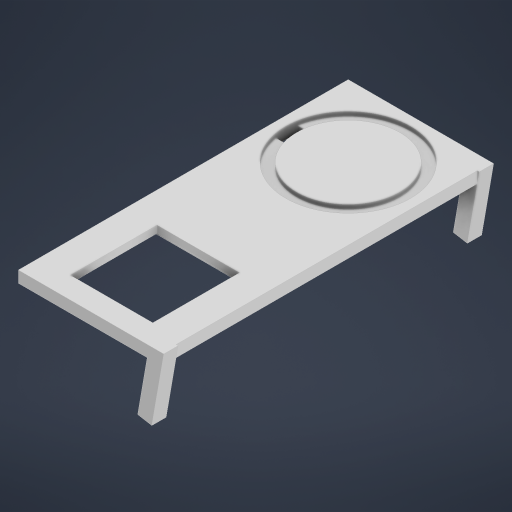
# Autodesk Inventor part: ViesCooleHouder
Saved by Autodesk Inventor 2023 (Build 270158000, 158)
## iProperties
Created: 2024-04-18
Part Number: ViesCooleHouder
Material: Generic
Document SubType Name: Modeling
Designer: warre
Density: 1 g/cm^3
Appearance: Default
Author: warre
Autodesk Inventor part; units mm, degrees
ref_plane "YZ Plane" through (0, 0, 0) normal (1, 0, 0) x (0, 1, 0)
ref_plane "XZ Plane" through (0, 0, 0) normal (0, 1, 0) x (-1, 0, 0)
ref_plane "XY Plane" through (0, 0, 0) normal (0, 0, 1) x (1, 0, 0)
sketch "Sketch1" plane through (0, 0, 0) normal (0, 1, 0) x (-1, 0, 0)
  line L0 (-50, 115) -> (50, 115)
  line L1 (50, 115) -> (50, -115)
  line L2 (50, -115) -> (-50, -115)
  line L3 (-50, -115) -> (-50, 115)
  line L4 (-50, 115) -> (50, -115) construction
  line L5 (50, 115) -> (-50, -115) construction
  circle A0 centre (0, -65) radius 43.5
  circle A1 centre (0, -65) radius 36
  line L6 (-28.75, 100) -> (28.75, 100)
  line L7 (28.75, 100) -> (28.75, 39.5)
  line L8 (28.75, 39.5) -> (-28.75, 39.5)
  line L9 (-28.75, 39.5) -> (-28.75, 100)
  line L10 (-28.75, 100) -> (28.75, 39.5) construction
  line L11 (28.75, 100) -> (-28.75, 39.5) construction
  point P0 (0, 0)
  point P1 (0, 69.75)
  dimension "d0" = 7.5
  dimension "d1" = 72
  dimension "d2" = 60.5
  dimension "d3" = 57.5
  dimension "d4" = 100
  dimension "d5" = 230
  dimension "d6" = 15
  dimension "d7" = 50
  constraints: 24 end point, 4 midpoint, 4 parallel, 2 centre point, 2 horizontal, 2 perpendicular, 2 vertical alignment, 1 coincident
  measures "d0" radial gap between concentric circles of A0 A1
  measures "d1" diameter of A1
  measures "d2" distance of L6.end L7.end
  measures "d3" distance between parallel lines of L9 L7
  measures "d4" distance between parallel lines of L3 L1
  measures "d5" distance of L2.end L0.start
  measures "d6" distance between parallel lines of L0 L6
  measures "d7" distance from line of L2 A0.centre
extrude "Extrusion1" add sketch "Sketch1" along normal blind 8
extrude "Extrusion2" add sketch "Sketch1" along normal blind 5 contours A0
sketch "Sketch2" plane through (0, 0, 0) normal (0, -1, 0) x (1, 0, 0)
  line L0 (50, -115) -> (-50, -115) projected
  line L1 (50, 115) -> (50, -115) projected
  line L2 (-50, 115) -> (50, 115) projected
  line L3 (-50, -115) -> (-50, 115) projected
  line L4 (28.75, 100) -> (-28.75, 100) projected
  line L5 (28.75, 39.5) -> (28.75, 100) projected
  line L6 (-28.75, 39.5) -> (28.75, 39.5) projected
  line L7 (-28.75, 100) -> (-28.75, 39.5) projected
  line L8 (-36.25, 37.25) -> (32.75, 37.25)
  line L9 (32.75, 37.25) -> (32.75, 102.25)
  line L10 (32.75, 102.25) -> (-36.25, 102.25)
  line L11 (-36.25, 102.25) -> (-36.25, 37.25)
  line L12 (-36.25, 37.25) -> (32.75, 102.25) construction
  line L13 (32.75, 37.25) -> (-36.25, 102.25) construction
  point P0 (0, 0)
  point P1 (-1.75, 69.75)
  dimension "d12" = 69
  dimension "d13" = 65
  dimension "d14" = 4
  dimension "d15" = 2.25
  constraints: 12 end point, 2 midpoint, 2 parallel, 1 horizontal, 1 perpendicular
  measures "d12" distance of L10.end L9.end
  measures "d13" distance of L9.end L8.end
  measures "d14" distance between parallel lines of L5 L9
  measures "d15" distance between parallel lines of L10 L4
extrude "Extrusion3" cut sketch "Sketch2" against normal blind 3 contours L11 L10 L9 L8
sketch "Sketch3" plane through (0, 5, -65) normal (0, 1, 0) x (1, 0, 0)
  circle A0 centre (0, 0) radius 36 projected
  circle A1 centre (0, 0) radius 43.5 projected
  circle A2 centre (0, 0) radius 43.5 projected
  circle A3 centre (0, 0) radius 36 projected
  circle A4 centre (0, 0) radius 36 projected
  line L0 (50, 50) -> (-50, 50) projected
  line L1 (-50, 50) -> (-50, -180) projected
  line L2 (-50, -180) -> (50, -180) projected
  line L3 (50, -180) -> (50, 50) projected
  line L4 (28.75, -165) -> (-28.75, -165) projected
  line L5 (-28.75, -165) -> (-28.75, -104.5) projected
  line L6 (-28.75, -104.5) -> (28.75, -104.5) projected
  line L7 (28.75, -104.5) -> (28.75, -165) projected
  circle A5 centre (0, 0) radius 43.5 projected
  line L8 (-35.2101, 7.5) -> (-42.8486, 7.5)
  line L9 (-42.8486, -7.5) -> (-35.2101, -7.5)
  point P0 (0, -65)
  point P1 (-39.0293, -7.5)
  point P2 (-35.2101, 7.5)
  point P3 (-42.8486, 7.5)
  dimension "d18" = 15
  constraints: 4 end point, 4 point on circle, 1 horizontal, 1 midpoint, 1 parallel, 1 vertical alignment
  measures "d18" distance from line of point (-39.029, -7.5) L8
extrude "Extrusion4" cut sketch "Sketch3" against normal through all contours A0 L9 A1 L8 picked at (-37.9902, -5.8388)
sketch "Sketch4" plane through (0, 0, 0) normal (0, -1, 0) x (1, 0, 0)
  arc A0 (-35.2101, -72.5) -> (-35.2101, -57.5) centre (0, -65) ccw projected
  arc A1 (-42.8486, -72.5) -> (-42.8486, -57.5) centre (0, -65) ccw projected
  line L0 (-30.5, -45) -> (30.5, -45)
  line L1 (30.5, -45) -> (30.5, -85)
  line L2 (30.5, -85) -> (-30.5, -85)
  line L3 (-30.5, -85) -> (-30.5, -45)
  line L4 (-30.5, -45) -> (30.5, -85) construction
  line L5 (30.5, -45) -> (-30.5, -85) construction
  point P0 (0, 0)
  point P1 (-30.5, -45.8754)
  point P2 (-30.5, -84.1246)
  point P3 (-29.9333, -85)
  point P4 (29.9333, -85)
  point P5 (30.5, -84.1246)
  point P6 (30.5, -45.8754)
  point P7 (29.9333, -45)
  point P8 (-29.9333, -45)
  dimension "d21" = 40
  dimension "d22" = 61
  constraints: 12 end point, 2 midpoint, 2 parallel, 1 horizontal, 1 perpendicular
  measures "d21" distance of L0.end L1.end
  measures "d22" distance of L1.end L2.end
extrude "Extrusion5" cut sketch "Sketch4" against normal blind 2 contours L3 A0 L0 L1 L2
sketch "Sketch5" plane through (0, 2, 0) normal (0, -1, 0) x (1, 0, 0)
  line L0 (-30.5, -84.1246) -> (-30.5, -45.8754) projected
  line L1 (-30.5, -45.8754) -> (-22.5, -45.8754)
  line L2 (-22.5, -45.8754) -> (-22.5, -84.1246)
  line L3 (-22.5, -84.1246) -> (-30.5, -84.1246)
  line L4 (-30.5, -84.1246) -> (-30.5, -45.8754)
  point P0 (0, 0)
  point P1 (-26.5, -84.1246)
  dimension "d25" = 8
  constraints: 8 end point, 2 parallel, 1 horizontal, 1 horizontal alignment, 1 midpoint, 1 perpendicular
  measures "d25" distance between parallel lines of L0 L2
extrude "Extrusion6" cut sketch "Sketch5" against normal blind 1
sketch "Sketch6" plane through (0, 0, 0) normal (0, -1, 0) x (1, 0, 0)
  circle A0 centre (-25.4, 20.875) radius 1.25
  circle A1 centre (-26.7, -28.625) radius 1.25
  circle A2 centre (24.1, -23.525) radius 1.25
  circle A3 centre (24.1, 6.375) radius 1.25
  line L0 (-29.9333, -45) -> (29.9333, -45) projected
  line L1 (32.75, 37.25) -> (-36.25, 37.25) projected
  point P0 (0, 0)
  point P1 (-25.4, -3.875)
  dimension "d28" = 2.5
  dimension "d29" = 2.5
  dimension "d30" = 2.5
  dimension "d31" = 2.5
  dimension "d32" = 29.9
  dimension "d33" = 1.3
  dimension "d34" = 50.8
  dimension "d35" = 49.5
  dimension "d36" = 5.1
  dimension "d37" = 24.75
  dimension "d38" = 82.25
  dimension "d39" = 41.125
  dimension "d40" = 25.4
  constraints: 4 centre point, 2 vertical alignment
  measures "d28" diameter of A0
  measures "d29" diameter of A1
  measures "d30" diameter of A2
  measures "d31" diameter of A3
  measures "d32" distance of A2.centre A3.centre
  measures "d33" horizontal distance of A0.centre A1.centre
  measures "d34" horizontal distance of A2.centre A1.centre
  measures "d35" vertical distance of A1.centre A0.centre
  measures "d36" vertical distance of A1.centre A2.centre
  measures "d37" distance of point (-25.4, -3.875) A0.centre
  measures "d38" distance between parallel lines of L0 L1
  measures "d39" distance from line of L1 point (-25.4, -3.875)
  measures "d40" horizontal distance of point (0, 0) point (-25.4, -3.875)
extrude "Extrusion7" add sketch "Sketch6" along normal blind 5
sketch "Sketch7" plane through (0, 0, 0) normal (0, -1, 0) x (1, 0, 0)
  line L0 (-36.25, 37.25) -> (-36.25, 102.25) projected
  line L1 (-36.25, 96.25) -> (-42.25, 96.25)
  line L2 (-42.25, 96.25) -> (-42.25, 43.25)
  line L3 (-42.25, 43.25) -> (-36.25, 43.25)
  line L4 (-36.25, 43.25) -> (-36.25, 96.25)
  line L5 (-36.25, 102.25) -> (32.75, 102.25) projected
  line L6 (32.75, 37.25) -> (-36.25, 37.25) projected
  point P0 (0, 0)
  point P1 (-39.25, 96.25)
  point P2 (-39.25, 43.25)
  dimension "d43" = 6
  dimension "d44" = 6
  dimension "d45" = 6
  constraints: 8 end point, 2 midpoint, 2 parallel, 1 horizontal, 1 perpendicular, 1 point on line
  measures "d43" distance from line of L5 point (-39.25, 96.25)
  measures "d44" distance from line of L6 point (-39.25, 43.25)
  measures "d45" distance between parallel lines of L0 L2
extrude "Extrusion8" cut sketch "Sketch7" against normal up to surface (3 mm away)
sketch "Sketch8" plane through (50, 0, -115) normal (0, 0, -1) x (-1, 0, 0)
  line L0 (0, 0) -> (0, 8) projected
  line L1 (0, 0) -> (6.9459, -39.3923)
  line L2 (6.9459, -39.3923) -> (16.794, -37.6558)
  line L3 (16.794, -37.6558) -> (10.1543, 0)
  line L4 (0, 0) -> (100, 0) projected
  line L5 (0, 0) -> (-1.4106, 8)
  line L6 (-1.4106, 8) -> (0, 8)
  point P0 (50, 0)
  dimension "d48" = 0
  dimension "d49" = 10
  dimension "d50" = 80
  dimension "d51" = 40
  constraints: 10 end point, 1 collinear, 1 horizontal, 1 perpendicular, 1 point on line
  measures "d48" angle of L1 L3
  measures "d49" distance of L1.end L2.end
  measures "d50" angle of L4 L1
  measures "d51" distance of L0.start L1.end
extrude "Extrusion9" add sketch "Sketch8" against normal blind 10
sketch "Sketch9" plane through (-50, 0, 115) normal (0, 0, 1) x (1, 0, 0)
  line L0 (89.8457, 0) -> (83.206, -37.6558) projected
  line L1 (83.206, -37.6558) -> (93.0541, -39.3923) projected
  line L2 (93.0541, -39.3923) -> (100, 0) projected
  line L3 (89.8457, 0) -> (100, 0) projected
  line L4 (101.4106, 8) -> (100, 8) projected
  line L5 (100, 0) -> (100, 8) projected
  line L6 (100, 0) -> (101.4106, 8) projected
  point P0 (50, 0)
extrude "Extrusion10" add sketch "Sketch9" against normal blind 10
body "Solid1"
